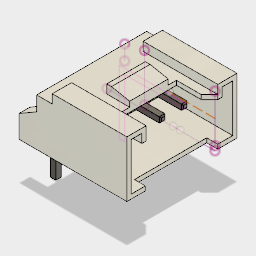
grove_female_angle v4 (Autodesk Fusion 360 design; units mm, degrees)
Autodesk Fusion 360 part; units mm, degrees
sketch "Sketch1" plane through (0, 0, 0) normal (0, 0, 1) x (1, 0, 0)
  line L0 (0, 0) -> (9.8, 0)
  line L1 (9.8, 0) -> (9.8, 5.1)
  line L2 (9.8, 5.1) -> (0, 5.1)
  line L3 (0, 5.1) -> (0, 0)
  dimension "d1" = 9.8
  dimension "d2" = 5.1
  measures "d1" distance of L0.start L0.end
  measures "d2" distance of L0.start L2.end
extrude "Extrude1" add sketch "Sketch1" along normal blind 10 makes body 1
sketch "Sketch2" plane through (0, 5.1, 0) normal (0, 1, 0) x (-1, 0, 0)
  line L0 (-9.8, 0) -> (0, 0)
  line L1 (0, 0) -> (0, 10)
  line L2 (0, 10) -> (-9.8, 10)
  line L3 (-9.8, 10) -> (-9.8, 0)
  line L4 (0, 5) -> (-9.8, 5) construction
  line L5 (-1.6, 5) -> (-1.6, 1)
  line L6 (-1.6, 1) -> (0, 1)
  line L7 (0, 9) -> (0, 1)
  line L8 (-1.6, 9) -> (0, 9)
  line L9 (-1.6, 5) -> (-1.6, 9)
  dimension "d5" = 8.2
  measures "d5" distance of L3 L5
extrude "Extrude2" cut sketch "Sketch2" against normal through all contours L1 L5 L6 L7 L8 L9 bodies 1
sketch "Sketch3" plane through (9.8, 0, 0) normal (1, 0, 0) x (0, 0, -1)
  line L0 (0, 0) -> (0, 5.1)
  line L1 (0, 5.1) -> (-10, 5.1)
  line L2 (-10, 5.1) -> (-10, 0)
  line L3 (-10, 0) -> (0, 0)
  line L4 (-5, 5.1) -> (-5, 0) construction
  line L5 (-5, 5.1) -> (-3.25, 5.1) construction
  line L6 (-5, 0) -> (-1.75, 0) construction
  line L7 (-3.25, 5.1) -> (-1.75, 5.1)
  line L8 (-1.75, 5.1) -> (-1.75, 4.3)
  line L9 (-1.75, 4.3) -> (-3.25, 4.3)
  line L10 (-3.25, 4.3) -> (-3.25, 5.1)
  line L11 (-6.75, 4.3) -> (-6.75, 5.1)
  line L12 (-8.25, 4.3) -> (-6.75, 4.3)
  line L13 (-6.75, 5.1) -> (-8.25, 5.1)
  line L14 (-8.25, 5.1) -> (-8.25, 4.3)
  dimension "d7" = 1.75
  dimension "d8" = 3.25
  dimension "d9" = 4.3
  measures "d7" distance of L4.start L5.end
  measures "d8" distance of L4.end L6.end
  measures "d9" distance of L3 L9
extrude "Extrude3" cut sketch "Sketch3" against normal through all contours L1 L7 L8 L9 L10 | L1 L11 L12 L13 L14 bodies 1
sketch "Sketch4" plane through (0, 0, 10) normal (0, 0, 1) x (1, 0, 0)
  line L0 (0, 5.1) -> (0, 0)
  line L1 (0, 0) -> (9.8, 0)
  line L2 (9.8, 0) -> (9.8, 5.1)
  line L3 (9.8, 5.1) -> (0, 5.1)
  line L4 (0, 2.0399) -> (1.6, 2.9637)
  line L5 (1.6, 2.9637) -> (1.6, 4.3)
  line L6 (1.6, 4.3) -> (3.0215, 4.3)
  line L7 (3.0215, 4.3) -> (3.0215, 5.1)
  line L8 (0, 5.1) -> (3.0215, 5.1)
  line L9 (0, 5.1) -> (0, 2.0399)
  line L10 (1.6, 5.1) -> (1.6, 0)
  dimension "d11" = 4.3
  dimension "d12" = 8.2
  dimension "d13" = 60
  measures "d11" distance of L1 L6
  measures "d12" distance of L2 L5
  measures "d13" angle of L4 L9
extrude "Extrude4" cut sketch "Sketch4" against normal through all contours L0 L3 L4 L5 L8 L9 L10 | L3 L6 L7 L8 L10 bodies 1
sketch "Sketch5" plane through (0, 5.1, 0) normal (0, 1, 0) x (-1, 0, 0)
  line L0 (-3.0215, 3.25) -> (-3.0215, 6.75)
  line L1 (-3.0215, 6.75) -> (-9.8, 6.75)
  line L2 (-9.8, 6.75) -> (-9.8, 3.25)
  line L3 (-9.8, 3.25) -> (-3.0215, 3.25)
  line L4 (-9.05, 2.5) -> (-6.8, 2.5)
  line L5 (-6.8, 2.5) -> (-6.8, 7.5)
  line L6 (-6.8, 7.5) -> (-9.05, 7.5)
  line L7 (-9.8, 7.5) -> (-9.8, 2.5)
  line L8 (-9.8, 1.75) -> (-9.8, 3.25)
  line L9 (-9.8, 1.75) -> (-9.05, 2.5)
  line L10 (-9.8, 1.75) -> (-8.7393, 1.75) construction
  line L11 (-9.8, 2.5) -> (-9.8, 1.75)
  line L12 (-9.8, 7.5) -> (-9.8, 8.25)
  line L13 (-9.8, 8.25) -> (-9.05, 7.5)
  point P0 (-9.8, 8.25)
  dimension "d15" = 0.75
  dimension "d16" = 0.75
  dimension "d17" = 3
  dimension "d18" = 45
  dimension "d19" = 45
  measures "d15" distance of L3 L4
  measures "d16" distance of L1 L6
  measures "d17" distance of L7.end L4.end
  measures "d18" angle of L9 L10
  measures "d19" angle of L12 L13
sketch "Sketch6" plane through (9.8, 0, 0) normal (1, 0, 0) x (0, 0, -1)
  line L0 (-8.25, 4.3) -> (-8.25, 5.1)
  line L1 (-8.25, 5.1) -> (-10, 5.1)
  line L2 (-10, 5.1) -> (-10, 0)
  line L3 (-10, 0) -> (0, 0)
  line L4 (0, 0) -> (0, 5.1)
  line L5 (0, 5.1) -> (-1.75, 5.1)
  line L6 (-1.75, 5.1) -> (-1.75, 4.3)
  line L7 (-1.75, 4.3) -> (-3.25, 4.3)
  line L8 (-3.25, 4.3) -> (-3.25, 5.1)
  line L9 (-3.25, 5.1) -> (-6.75, 5.1)
  line L10 (-6.75, 5.1) -> (-6.75, 4.3)
  line L11 (-6.75, 4.3) -> (-8.25, 4.3)
  line L12 (-9.6, 0.4) -> (-0.4, 0.4)
  line L13 (-0.4, 0.4) -> (-0.4, 4.7)
  line L14 (-0.4, 4.7) -> (-1.35, 4.7)
  line L15 (-1.35, 4.7) -> (-1.35, 3.9)
  line L16 (-1.35, 3.9) -> (-3.65, 3.9)
  line L17 (-3.65, 3.9) -> (-3.65, 4.7) construction
  line L18 (-3.65, 4.7) -> (-6.35, 4.7) construction
  line L19 (-6.35, 4.7) -> (-6.35, 3.9) construction
  line L20 (-6.35, 3.9) -> (-8.65, 3.9)
  line L21 (-8.65, 3.9) -> (-8.65, 4.7)
  line L22 (-8.65, 4.7) -> (-9.6, 4.7)
  line L23 (-9.6, 4.7) -> (-9.6, 0.4)
  line L24 (-6.35, 3.9) -> (-3.65, 3.9)
  dimension "d20" = 0.4
extrude "Extrude5" cut sketch "Sketch6" against normal blind 6.4 contours L12 L13 L14 L15 L16 L20 L21 L22 L23 L24 bodies 1
extrude "Extrude6" cut sketch "Sketch5" against normal up to surface (1.2 mm away) contours L3 L4 L5 L7 L8 L9 L11 | L1 L2 L3 L5 L7 | L1 L5 L6 L7 L12 L13 bodies 1
extrude "Extrude7" cut 1 faces at (3.0215, 4.5667, 5.5833) along direction (1, 0, 0) blind 1.7 on bodies 1 bodies 1
sketch "Sketch8" plane through (0, 0, 6.75) normal (0, 0, 1) x (1, 0, 0)
  line L0 (4.7215, 5.1) -> (4.7215, 4.3)
  line L1 (4.7215, 4.3) -> (6.8, 4.3)
  line L2 (6.8, 4.3) -> (6.8, 5.1)
  line L3 (6.8, 5.1) -> (4.7215, 5.1)
  line L4 (6.8, 4.7785) -> (5.1492, 5.1)
  line L5 (6.8, 5.1) -> (5.1492, 5.1)
  line L6 (6.8, 4.7785) -> (6.8, 5.1)
extrude "Extrude8" cut sketch "Sketch8" against normal up to surface (3.5 mm away) contours L2 L3 L4 L5 L6 bodies 1
sketch "Sketch9" plane through (9.8, 0, 0) normal (1, 0, 0) x (0, 0, -1)
  line L0 (-1.75, 4.3) -> (-1.75, 3.9)
  line L1 (-1.75, 3.9) -> (-1.35, 3.9)
  line L2 (-1.35, 3.9) -> (-1.35, 4.7)
  line L3 (-1.35, 4.7) -> (-0.4, 4.7)
  line L4 (-0.4, 4.7) -> (-0.4, 0.4)
  line L5 (-0.4, 0.4) -> (-9.6, 0.4)
  line L6 (-9.6, 0.4) -> (-9.6, 4.7)
  line L7 (-9.6, 4.7) -> (-8.65, 4.7)
  line L8 (-8.65, 4.7) -> (-8.65, 3.9)
  line L9 (-8.65, 3.9) -> (-8.25, 3.9)
  line L10 (-8.25, 3.9) -> (-8.25, 4.3)
  line L11 (-8.25, 4.3) -> (-8.25, 5.1)
  line L12 (-8.25, 5.1) -> (-10, 5.1)
  line L13 (-10, 5.1) -> (-10, 0)
  line L14 (-10, 0) -> (0, 0)
  line L15 (0, 0) -> (0, 5.1)
  line L16 (0, 5.1) -> (-1.75, 5.1)
  line L17 (-1.75, 5.1) -> (-1.75, 4.3)
  line L18 (-8.3174, 0.4) -> (-1.75, 0.4)
  line L19 (-1.75, 0.4) -> (-1.75, 0)
  line L20 (-1.75, 0) -> (-8.3174, 0)
  line L21 (-8.3174, 0) -> (-8.3174, 0.4)
extrude "Extrude9" cut sketch "Sketch9" against normal blind 1 contours L5 L14 L18 L19 L20 L21 bodies 1
ref_plane "WorkPlane1" through (4.9, 2.55, 5) normal (0, 0, 1) x (1, 0, 0)
ref_plane "WorkPlane2" through (4.9, 2.55, 2) normal (0, 0, 1) x (1, 0, 0)
sketch "Sketch10" plane through (4.9, 2.55, 2) normal (0, 0, 1) x (1, 0, 0)
  line L0 (4.9, 2.15) -> (4.9, -2.15)
  line L1 (-1.5, 2.15) -> (-1.5, -2.15)
  line L2 (4.9, 0) -> (0.8, 0) construction
  line L3 (1.1, -2.5) -> (1.7485, -2.5)
  line L4 (-3.3, -0.15) -> (-3.8, -0.15)
  line L5 (-3.8, -0.15) -> (-3.8, -5.95)
  line L6 (-3.8, -5.95) -> (-3.3, -5.95)
  line L7 (-3.3, -5.95) -> (-3.3, -0.65)
  line L8 (-3.3, 1.75) -> (-3.3, 0.4137)
  line L9 (-3.3, -0.15) -> (2.2, -0.15)
  line L10 (2.2, -0.15) -> (2.2, -0.65)
  line L11 (2.2, -0.65) -> (-3.3, -0.65)
  line L12 (-4.9, -2.55) -> (4.9, -2.55)
  dimension "d33" = 0.5
  dimension "d34" = 0.5
  dimension "d35" = 3.4
  dimension "d40" = 1.9
  dimension "d41" = 5.5
  measures "d33" distance of L4.start L4.end
  measures "d34" distance of L4.start L7.end
  measures "d35" distance of L6 L12
  measures "d40" distance of L11 L12
  measures "d41" distance of L7 L10
copy_body "Body->Comp1" bodies 1 removing the originals makes body 2 in component "housing"
extrude "Extrude1'" add sketch "Sketch10" along normal mid plane 0.5 separate body makes body 3 in component "Component"
chamfer "Chamfer1" distance 0.1 angle 45 4 edges at (7.1, 2.4, 2) (7.1, 2.15, 2.25) (7.1, 1.9, 2) (7.1, 2.15, 1.75) on bodies 3 in component "Component"
chamfer "Chamfer2" distance 0.1 angle 45 4 edges at (1.35, -3.4, 2.25) (1.6, -3.4, 2) (1.35, -3.4, 1.75) (1.1, -3.4, 2) on bodies 3 in component "Component"
pattern_linear "R-Pattern1" count 4 spacing 2 along (0, 0, 1) of bodies 3 makes body 4 at (3.2333, 2.2333, 3.75) makes body 5 at (3.2333, 2.2333, 5.75) makes body 6 at (3.2333, 2.2333, 7.75) in component "Component"
component "housing" placed x (1, 0, 0) y (0, 1, 0) z (0, 0, 1) at (0, 0, 0)
component "Component" placed x (1, 0, 0) y (0, 1, 0) z (0, 0, 1) at (0, 0, 0)
equation "d7 = ( 3.5 / 2 ) * 1 mm"
equation "d8 = 3 mm + ( ( 0.5 / 2 ) * 1 mm )"
equation "d40 = 2.15 mm - 0.25 mm"
